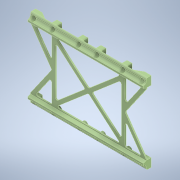
# Autodesk Inventor part: BodyStructure Centre
Saved by Autodesk Inventor 2022.2 (Build 262287030, 287C)
## iProperties
Created: 2019-11-07
Part Number: BodyStructure Centre
Material: solidworks materials|ABS
Document SubType Name: Modeling
Designer: Jochen
Density: 1.02 g/cm^3
Appearance: 151,157,178
Sending System: SolidWorks 2017
Last Author: Felix
Last Saved: 2021-02-23
Author: Jochen
Autodesk Inventor part; units mm, degrees
ref_plane "YZ Plane" through (0, 0, 0) normal (1, 0, 0) x (0, 1, 0)
ref_plane "XZ Plane" through (0, 0, 0) normal (0, 1, 0) x (-1, 0, 0)
ref_plane "Work Plane1" through (0, 0, 30) normal (0, 0, 1) x (1, 0, 0)
sketch "Sketch1" plane through (0, 0, 30) normal (0, 0, 1) x (1, 0, 0)
  line L0 (-80, -55) -> (80, -55)
  line L1 (80, 55) -> (-80, 55)
  line L2 (80, 42) -> (80, 42)
  line L3 (0, -77.5799) -> (0, 77.5799) construction
  line L4 (-112, 0) -> (112, 0) construction
  line L5 (-50.649, -42) -> (-50.649, -8.7287)
  line L6 (-45.649, 35.4185) -> (-45.649, -35.4185)
  line L7 (-50.649, -8.7287) -> (-73.9001, -42)
  line L8 (-80, -42) -> (-50.649, 0)
  line L9 (50.649, -8.7287) -> (73.9001, -42)
  line L10 (50.649, -42) -> (50.649, -8.7287)
  line L11 (45.649, 35.4185) -> (45.649, -35.4185)
  line L12 (80, -42) -> (50.649, 0)
  line L13 (50.649, 8.7287) -> (73.9001, 42)
  line L14 (80, 42) -> (50.649, 0)
  line L15 (50.649, 0) -> (50.649, 0)
  line L16 (50.649, 8.7287) -> (50.649, 42)
  line L17 (-50.649, 0) -> (-50.649, 0)
  line L18 (-80, 42) -> (-50.649, 0)
  line L19 (-50.649, 8.7287) -> (-73.9001, 42)
  line L20 (-80, 42) -> (-80, 42)
  line L21 (-50.649, 8.7287) -> (-50.649, 42)
  line L22 (73.9001, 42) -> (50.649, 42)
  line L23 (-73.9001, 42) -> (-50.649, 42)
  line L24 (-45.649, 42) -> (45.649, 42)
  line L25 (-80, -42) -> (-80, -42)
  line L26 (-50.649, -42) -> (-73.9001, -42)
  line L27 (45.649, -42) -> (-45.649, -42)
  line L28 (80, -42) -> (80, -42)
  line L29 (73.9001, -42) -> (50.649, -42)
  line L30 (80, -55) -> (80, -42)
  line L31 (80, 42) -> (80, 55)
  line L32 (-80, 55) -> (-80, 42)
  line L33 (-80, -42) -> (-80, -55)
  line L34 (-48.149, 55) -> (-48.149, -55) construction
  line L35 (-45.649, 42) -> (0, 2.9266)
  line L36 (0, 2.9266) -> (45.649, 42)
  line L37 (45.649, 35.4185) -> (4.2699, 0)
  line L38 (45.649, -35.4185) -> (4.2699, 0)
  line L39 (0, -2.9266) -> (45.649, -42)
  line L40 (-4.2699, 0) -> (-45.649, 35.4185)
  line L41 (-4.2699, 0) -> (-45.649, -35.4185)
  line L42 (0, -2.9266) -> (-45.649, -42)
  point P0 (0, 0)
  point P1 (-2.5, 42)
  point P2 (2.5, 42)
  point P3 (2.5, -42)
  point P4 (-2.5, -42)
  point P5 (50.649, 0)
  point P6 (-50.649, 0)
  dimension "d2" = 5
  dimension "d3" = 0
  dimension "d4" = 160
  dimension "d5" = 13
  dimension "d7" = 110
  dimension "d101" = 5
  dimension "d107" = 5
  constraints: 82 end point, 17 parallel, 15 collinear, 15 perpendicular, 11 point on line, 9 horizontal, 2 vertical, 19 other
  measures "d2" distance between parallel lines of L6 L5
  measures "d3" distance of L8.start L25.end
  measures "d4" distance of L0.start L0.end
  measures "d5" distance of L25.end L0.start
  measures "d7" distance between parallel lines of L1 L0
  measures "d101" distance between parallel lines of L8 L7
  measures "d107" distance between parallel lines of L42 L41
extrude "Extrusion1" add sketch "Sketch1" along normal blind 15.5
fillet "Fillet1" radius 2 22 edges at (-50.649, -42, 37.75) (-50.649, -8.7287, 37.75) (-73.9001, -42, 37.75) (-73.9001, 42, 37.75) (-50.649, 42, 37.75) (-50.649, 8.7287, 37.75) (50.649, -8.7287, 37.75) (50.649, -42, 37.75) (50.649, 42, 37.75) (50.649, 8.7287, 37.75) (73.9001, 42, 37.75) (73.9001, -42, 37.75) (-45.649, 35.4185, 37.75) (0, -2.9266, 37.75) (4.2699, 0, 37.75) (0, 2.9266, 37.75) (-4.2699, 0, 37.75) (-45.649, -35.4185, 37.75) (45.649, -35.4185, 37.75) (45.649, 35.4185, 37.75) (50.649, 0, 37.75) (-50.649, 0, 37.75)
fillet "Fillet1" radius 2 4 edges at (-45.649, 42, 37.75) (-45.649, -42, 37.75) (45.649, -42, 37.75) (45.649, 42, 37.75)
sketch "Sketch3" plane through (0, 0, 0) normal (1, 0, 0) x (0, 1, 0)
  line L0 (0, -10.1) -> (0, 60.6) construction
  line L1 (-77.5799, 0) -> (77.5799, 0) construction
  line L2 (-42, 45.5) -> (-55, 45.5) construction
  line L3 (-55, 45.5) -> (-42, 45.5) construction
  line L4 (-42, 45.5) -> (-1.1456, 45.5) construction
  line L5 (1.1456, 45.5) -> (42, 45.5) construction
  line L6 (42, 45.5) -> (55, 45.5) construction
  line L7 (55, 45.5) -> (42, 45.5) construction
  line L8 (42, 45.5) -> (1.1456, 45.5) construction
  line L9 (-1.1456, 45.5) -> (-42, 45.5) construction
  line L10 (13.9365, 45.5) -> (38.8544, 45.5) construction
  line L11 (42, 45.5) -> (38.8544, 45.5) construction
  line L12 (40, 45.5) -> (42, 45.5) construction
  line L13 (40, 45.5) -> (15.0821, 45.5) construction
  line L14 (13.9365, 45.5) -> (15.0821, 45.5) construction
  line L15 (15.0821, 45.5) -> (40, 45.5) construction
  line L16 (42, 45.5) -> (40, 45.5) construction
  line L17 (38.8544, 45.5) -> (42, 45.5) construction
  line L18 (38.8544, 45.5) -> (13.9365, 45.5) construction
  line L19 (15.0821, 45.5) -> (13.9365, 45.5) construction
  line L20 (-13.9365, 45.5) -> (-38.8544, 45.5) construction
  line L21 (-40, 45.5) -> (-42, 45.5) construction
  line L22 (-40, 45.5) -> (-15.0821, 45.5) construction
  line L23 (-13.9365, 45.5) -> (-15.0821, 45.5) construction
  line L24 (-38.8544, 45.5) -> (-42, 45.5) construction
  line L25 (-38.8544, 45.5) -> (-13.9365, 45.5) construction
  line L26 (-15.0821, 45.5) -> (-13.9365, 45.5) construction
  line L27 (-15.0821, 45.5) -> (-40, 45.5) construction
  line L28 (-42, 45.5) -> (-40, 45.5) construction
  line L29 (-42, 30) -> (-55, 30) construction
  line L30 (-1.1456, 30) -> (-42, 30) construction
  line L31 (42, 30) -> (1.1456, 30) construction
  line L32 (55, 30) -> (42, 30) construction
  line L33 (42, 30) -> (55, 30) construction
  line L34 (1.1456, 30) -> (42, 30) construction
  line L35 (-42, 30) -> (-1.1456, 30) construction
  line L36 (-55, 30) -> (-42, 30) construction
  line L37 (15.0821, 30) -> (13.9365, 30) construction
  line L38 (40, 30) -> (15.0821, 30) construction
  line L39 (42, 30) -> (40, 30) construction
  line L40 (38.8544, 30) -> (42, 30) construction
  line L41 (13.9365, 30) -> (38.8544, 30) construction
  line L42 (13.9365, 30) -> (15.0821, 30) construction
  line L43 (38.8544, 30) -> (13.9365, 30) construction
  line L44 (42, 30) -> (38.8544, 30) construction
  line L45 (40, 30) -> (42, 30) construction
  line L46 (15.0821, 30) -> (40, 30) construction
  line L47 (-15.0821, 30) -> (-13.9365, 30) construction
  line L48 (-40, 30) -> (-15.0821, 30) construction
  line L49 (-42, 30) -> (-40, 30) construction
  line L50 (-13.9365, 30) -> (-38.8544, 30) construction
  line L51 (-40, 30) -> (-42, 30) construction
  line L52 (-15.0821, 30) -> (-40, 30) construction
  line L53 (-13.9365, 30) -> (-15.0821, 30) construction
  line L54 (-38.8544, 30) -> (-13.9365, 30) construction
  line L55 (-42, 30) -> (-38.8544, 30) construction
  line L56 (55, 30) -> (55, 45.5) construction
  line L57 (55, 30) -> (55, 45.5) construction
  line L58 (-55, 30) -> (-55, 45.5) construction
  line L59 (-55, 30) -> (-55, 45.5) construction
  line L60 (-37, 30) -> (-37, 45.5) construction
  line L61 (-37, 30) -> (-37, 45.5) construction
  line L62 (-55, 30) -> (-55, 39.5)
  line L63 (-53, 41.5) -> (-48.9559, 41.5)
  line L64 (-48.9559, 41.5) -> (-47.5, 45.5)
  line L65 (-47.5, 45.5) -> (-45, 45.5)
  line L66 (-45, 45.5) -> (-43.5441, 41.5)
  line L67 (-43.5441, 41.5) -> (43.5441, 41.5)
  line L68 (43.5441, 41.5) -> (45, 45.5)
  line L69 (45, 45.5) -> (47.5, 45.5)
  line L70 (47.5, 45.5) -> (48.9559, 41.5)
  line L71 (55, 39.5) -> (55, 30)
  line L72 (55, 30) -> (-55, 30)
  line L73 (-46.25, 45.5) -> (-46.25, 30) construction
  line L74 (53, 41.5) -> (48.9559, 41.5)
  arc A0 (-53, 41.5) -> (-55, 39.5) centre (-53, 39.5) ccw
  arc A1 (55, 39.5) -> (53, 41.5) centre (53, 39.5) ccw
  line L75 (-38.8544, 30) -> (-42, 30) projected
  line L76 (-42, 45.5) -> (-38.8544, 45.5) projected
  line L77 (-47.5, 50.5) -> (-45, 50.5)
  line L78 (-45, 50.5) -> (-43.5441, 41.5)
  line L79 (-48.9559, 41.5) -> (-47.5, 50.5)
  line L80 (42, 45.5) -> (42, 30) projected
  line L81 (42, 30) -> (42, 45.5) projected
  line L82 (1.1456, 30) -> (-1.1456, 30) projected
  line L83 (-1.1456, 30) -> (1.1456, 30) projected
  line L84 (1.1456, 45.5) -> (-1.1456, 45.5) projected
  line L85 (-1.1456, 45.5) -> (1.1456, 45.5) projected
  point P0 (0, 0)
  point P1 (-55, 34.75)
  point P2 (50, 33)
  point P3 (48, 35)
  point P4 (-46.25, 50.5)
  dimension "d28" = 110
  dimension "d29" = 2.5
  dimension "d30" = 4
  dimension "d37" = 10
  dimension "d38" = 2
  dimension "d84" = 5
  constraints: 32 end point, 7 point on line, 4 parallel, 4 point on circle, 4 tangent, 3 collinear, 3 midpoint, 3 perpendicular, 2 centre point, 2 horizontal, 1 equal radius, 1 vertical, 5 other
  measures "d28" angle of L64 L65
  measures "d29" distance of L64.end L65.end
  measures "d30" distance between parallel lines of L63 L65
  measures "d37" distance from line of L58 L65.end
  measures "d38" radius of A0
  measures "d84" distance from line of point (-46.25, 50.5) L2
extrude "Extrusion3" cut sketch "Sketch3" along normal through all both and the other way through all contours L62 A0 L63 L64 L65 L66 L67 L80 L72 | L80 L67 L68 L69 L70 L74 A1 L71 L72 keep common part
sketch "Sketch12" plane through (80, -55, 30) normal (1, 0, 0) x (0, 0, -1)
  arc A0 (-11.5, 2) -> (-9.5, 0) centre (-9.5, 2) ccw projected
  line L0 (-11.5, 2) -> (-11.5, 6.0441) projected
  line L1 (-11.5, 6.0441) -> (-15.5, 7.5) projected
  line L2 (-15.5, 7.5) -> (-15.5, 10) projected
  line L3 (-15.5, 10) -> (-11.5, 11.4559) projected
  line L4 (-11.5, 11.4559) -> (-11.5, 13) projected
  line L5 (0, 13) -> (0, 0) projected
  line L6 (0, 0) -> (-9.5, 0) projected
  line L7 (-11.5, 97) -> (-11.5, 98.5441) projected
  line L8 (-11.5, 98.5441) -> (-15.5, 100) projected
  line L9 (-15.5, 100) -> (-15.5, 102.5) projected
  line L10 (-15.5, 102.5) -> (-11.5, 103.9559) projected
  line L11 (-11.5, 103.9559) -> (-11.5, 108) projected
  arc A1 (-9.5, 110) -> (-11.5, 108) centre (-9.5, 108) ccw projected
  line L12 (-9.5, 110) -> (0, 110) projected
  line L13 (0, 110) -> (0, 97) projected
  line L14 (-11.5, 6.0441) -> (-11.5, 2) projected
  line L15 (-11.5, 6.0441) -> (-11.5, 11.4559)
  line L16 (-11.5, 98.5441) -> (-11.5, 103.9559)
  line L17 (-11.5, 13) -> (0, 13) projected
  line L18 (0, 97) -> (-11.5, 97) projected
  point P0 (30, 55)
  constraints: 4 end point, 2 collinear
sketch "Sketch5" plane through (0, 0, 0) normal (0, 1, 0) x (-1, 0, 0)
  line L0 (114, 0) -> (-124, 0) construction
  line L1 (0, -9.1) -> (0, 54.6) construction
  line L2 (80, 41.5) -> (80, 45.5) construction
  line L3 (80, 45.5) -> (-90, 45.5) construction
  line L4 (-80, 30) -> (-80, 39.5) construction
  line L5 (-80, 30) -> (80, 30) construction
  line L6 (80, 30) -> (80, 39.5) construction
  line L7 (80, 39.5) -> (80, 41.5) construction
  line L8 (-80, 41.5) -> (-80, 39.5) construction
  line L9 (80, 39.5) -> (-80, 39.5) construction
  line L10 (-71, 34.5) -> (-61.4737, 40)
  line L11 (-61.4737, 40) -> (-52, 40)
  line L12 (-52, 40) -> (-52, 33)
  line L13 (-52, 33) -> (-45, 33)
  line L14 (-45, 33) -> (-45, 40)
  line L15 (-45, 40) -> (-16, 40)
  line L16 (-16, 40) -> (-16, 33)
  line L17 (-16, 33) -> (-9, 33)
  line L18 (-9, 33) -> (-9, 40)
  line L19 (-9, 40) -> (9, 40)
  line L20 (9, 40) -> (9, 33)
  line L21 (9, 33) -> (16, 33)
  line L22 (16, 33) -> (16, 40)
  line L23 (16, 40) -> (45, 40)
  line L24 (45, 40) -> (45, 33)
  line L25 (45, 33) -> (52, 33)
  line L26 (52, 33) -> (52, 40)
  line L27 (52, 40) -> (61.4737, 40)
  line L28 (61.4737, 40) -> (71, 34.5)
  line L29 (80, 34.5) -> (80, 45.5)
  line L30 (80, 30) -> (-80, 30) construction
  line L31 (80, 45.5) -> (-90, 45.5)
  line L32 (-90, 45.5) -> (-90, 34.5)
  line L33 (80, 41.5) -> (-80, 41.5) projected
  line L34 (80, 39.5) -> (-80, 39.5) projected
  line L35 (71, 34.5) -> (80, 34.5)
  line L36 (-90, 34.5) -> (-71, 34.5)
  line L37 (52, 40) -> (45, 40) construction
  line L38 (80, 39.5) -> (-80, 39.5) construction
  line L39 (-80, 45.5) -> (80, 45.5) construction
  point P0 (0, 0)
  point P1 (56.7369, 40)
  point P2 (48.5, 33)
  dimension "d44" = 30
  dimension "d47" = 7
  dimension "d48" = 9
  dimension "d49" = 5.5
  dimension "d51" = 11
  dimension "d52" = 9
  dimension "d96" = 7
  dimension "d102" = 48.5
  constraints: 54 end point, 15 point on line, 11 perpendicular, 4 collinear, 4 parallel, 2 midpoint, 1 vertical, 4 other
  measures "d44" angle of L5 L28
  measures "d47" distance between parallel lines of L26 L24
  measures "d48" distance between parallel lines of L1 L20
  measures "d49" distance from line of L3 point (56.737, 40)
  measures "d51" distance from line of L2.end L35
  measures "d52" distance of L28.end L29.start
  measures "d96" distance between parallel lines of L25 L37
  measures "d102" distance from line of L1 point (48.5, 33)
extrude "Extrusion5" cut sketch "Sketch5" along normal through all both and the other way through all contours L36 L32 L31 L29 L34 L28 L27 L26 L24 L23 L22 L20 L19 L18 L16 L15 L14 L12 L11 L10 | L34 L14 L13 L12 | L34 L18 L17 L16 | L29 L35 L28 L34 | L34 L22 L21 L20 | L26 L25 L24 L34 keep common part
sketch "Sketch6" plane through (0, 0, 0) normal (1, 0, 0) x (0, 1, 0)
  line L0 (0, -9.1) -> (0, 54.6) construction
  line L1 (-77.5799, 0) -> (77.5799, 0) construction
  line L2 (-38.535, 41.5) -> (-36.9915, 41.5) construction
  line L3 (-46.25, 40) -> (-46.25, 25)
  line L4 (-46.25, 25) -> (46.25, 25)
  line L5 (46.25, 25) -> (46.25, 40)
  line L6 (-46.25, 40) -> (46.25, 40)
  line L7 (-54.9365, 40) -> (54.9365, 40) projected
  line L8 (-45, 45.5) -> (-47.5, 45.5) construction
  line L9 (46.25, 25) -> (53.5, 25)
  line L10 (53.5, 25) -> (53.5, 40)
  line L11 (46.25, 40) -> (53.5, 40)
  line L12 (-46.25, 40) -> (-53.5, 40)
  line L13 (-53.5, 40) -> (-53.5, 25)
  line L14 (-53.5, 25) -> (-46.25, 25)
  line L15 (55, 33) -> (55, 39.5) projected
  line L16 (55, 33) -> (55, 25)
  line L17 (55, 25) -> (53.5, 25)
  line L18 (55, 33) -> (55, 40)
  line L19 (55, 40) -> (53.5, 40)
  line L20 (-53.5, 25) -> (-55, 25)
  line L21 (-55, 25) -> (-55, 40)
  line L22 (-55, 40) -> (-53.5, 40)
  point P0 (0, 0)
  point P1 (-46.25, 32.5)
  point P2 (42, 40)
  point P3 (-46.25, 45.5)
  point P4 (-55, 33)
  dimension "d75" = 1.5
  dimension "d104" = 15
  dimension "d106" = 7.25
  constraints: 36 end point, 7 point on line, 6 perpendicular, 4 collinear, 2 horizontal, 2 midpoint, 2 vertical, 1 parallel, 1 other
  measures "d75" distance between parallel lines of L6 L2
  measures "d104" distance from line of L6 L3.end
  measures "d106" distance between parallel lines of L5 L10
extrude "Extrusion6" cut sketch "Sketch6" along normal mid plane 140 contours L6 L5 L4 L3
sketch "Sketch9" plane through (45, -54.9365, 40) normal (0, 0, -1) x (-1, 0, 0)
  line L0 (-25, 91.3557) -> (-9.2884, 68.873) projected
  arc A0 (-9.2884, 68.873) -> (-5.649, 70.0186) centre (-7.649, 70.0186) ccw projected
  arc A1 (-5.649, 94.9365) -> (-7.649, 96.9365) centre (-7.649, 94.9365) ccw projected
  line L1 (-7.649, 96.9365) -> (-25, 96.9365) projected
  line L2 (-6.4496, 56.0821) -> (-25, 82.6269) projected
  line L3 (-35, 96.9365) -> (-35, 109.873) projected
  line L4 (-25, 82.6269) -> (-35, 96.9365) projected
  line L5 (-25, 27.2461) -> (-6.4496, 53.7909) projected
  line L6 (-35, 0) -> (-35, 12.9365) projected
  line L7 (-35, 12.9365) -> (-25, 27.2461) projected
  line L8 (125, 96.9365) -> (115, 82.6269) projected
  line L9 (125, 109.873) -> (125, 96.9365) projected
  line L10 (115, 27.2461) -> (125, 12.9365) projected
  line L11 (125, 12.9365) -> (125, 0) projected
  arc A2 (-5.649, 39.8543) -> (-9.2884, 41) centre (-7.649, 39.8543) ccw projected
  line L12 (-9.2884, 41) -> (-25, 18.5173) projected
  line L13 (-25, 12.9365) -> (-7.649, 12.9365) projected
  arc A3 (-7.649, 12.9365) -> (-5.649, 14.9365) centre (-7.649, 14.9365) ccw projected
  circle A4 centre (-30, 104.9365) radius 1.5
  circle A5 centre (32.5, 104.9365) radius 1.5
  circle A6 centre (-3.5, 104.9365) radius 1.5
  circle A7 centre (57.5, 104.9365) radius 1.5
  circle A8 centre (93.5, 104.9365) radius 1.5
  circle A9 centre (120, 104.9365) radius 1.5
  circle A10 centre (120, 4.9365) radius 1.5
  circle A11 centre (93.5, 4.9365) radius 1.5
  circle A12 centre (57.5, 4.9365) radius 1.5
  circle A13 centre (-3.5, 4.9365) radius 1.5
  circle A14 centre (32.5, 4.9365) radius 1.5
  circle A15 centre (-30, 4.9365) radius 1.5
  line L14 (-30, 104.9365) -> (120, 104.9365) construction
  line L15 (120, 104.9365) -> (120, 4.9365) construction
  line L16 (120, 4.9365) -> (-30, 4.9365) construction
  line L17 (-30, 4.9365) -> (-30, 104.9365) construction
  line L18 (157, 54.9365) -> (-67, 54.9365) construction
  line L19 (45, -22.6434) -> (45, 132.5164) construction
  line L20 (32.5, 104.9365) -> (32.5, 4.9365) construction
  line L21 (-3.5, 4.9365) -> (-3.5, 104.9365) construction
  line L22 (93.5, 104.9365) -> (93.5, 4.9365) construction
  line L23 (57.5, 104.9365) -> (57.5, 4.9365) construction
  circle A16 centre (-30, 4.9365) radius 2.9
  circle A17 centre (-3.5, 4.9365) radius 2.9
  circle A18 centre (32.5, 4.9365) radius 2.9
  circle A19 centre (57.5, 4.9365) radius 2.9
  circle A20 centre (93.5, 4.9365) radius 2.9
  circle A21 centre (120, 4.9365) radius 2.9
  circle A22 centre (120, 104.9365) radius 2.9
  circle A23 centre (93.5, 104.9365) radius 2.9
  circle A24 centre (57.5, 104.9365) radius 2.9
  circle A25 centre (32.5, 104.9365) radius 2.9
  circle A26 centre (-3.5, 104.9365) radius 2.9
  circle A27 centre (-30, 104.9365) radius 2.9
  line L24 (125, 0) -> (106.4737, 0) projected
  line L25 (-35, 109.873) -> (-16.4737, 109.873) projected
  line L26 (106.4737, 109.873) -> (125, 109.873) projected
  line L27 (-16.4737, 0) -> (-35, 0) projected
  line L28 (116.7018, 16.0821) -> (115, 18.5173) projected
  line L29 (115, 91.3557) -> (116.7018, 93.7909) projected
  line L30 (-26.7018, 93.7909) -> (-25, 91.3557) projected
  line L31 (-25, 18.5173) -> (-26.7018, 16.0821) projected
  line L32 (-5.649, 14.9365) -> (-5.649, 39.8543) projected
  line L33 (61, 8.6865) -> (61, 0) projected
  line L34 (106.4737, 0) -> (106.4737, 8.6865) projected
  line L35 (115, 18.5173) -> (115, 27.2461) projected
  line L36 (-16.4737, 109.873) -> (-16.4737, 101.1865) projected
  line L37 (95.649, 39.8543) -> (95.649, 14.9365) projected
  line L38 (97, 109.873) -> (97, 101.1865) projected
  line L39 (90, 101.1865) -> (90, 109.873) projected
  line L40 (54, 101.1865) -> (54, 109.873) projected
  line L41 (36, 109.873) -> (36, 101.1865) projected
  line L42 (29, 101.1865) -> (29, 109.873) projected
  line L43 (0, 109.873) -> (0, 101.1865) projected
  line L44 (-7, 101.1865) -> (-7, 109.873) projected
  line L45 (96.4496, 53.7909) -> (115, 27.2461) projected
  line L46 (115, 82.6269) -> (96.4496, 56.0821) projected
  line L47 (99.2884, 68.873) -> (115, 91.3557) projected
  line L48 (97.649, 12.9365) -> (115, 12.9365) projected
  line L49 (115, 18.5173) -> (99.2884, 41) projected
  line L50 (-25, 27.2461) -> (-25, 18.5173) projected
  line L51 (-25.0624, 12.9365) -> (-25, 12.9365) projected
  arc A28 (-26.7018, 16.0821) -> (-25.0624, 12.9365) centre (-25.0624, 14.9365) ccw projected
  line L52 (-25, 8.6865) -> (-16.4737, 8.6865) projected
  line L53 (-25, 12.9365) -> (-25, 8.6865) projected
  line L54 (-25, 91.3557) -> (-25, 82.6269) projected
  arc A29 (-25.0624, 96.9365) -> (-26.7018, 93.7909) centre (-25.0624, 94.9365) ccw projected
  line L55 (-25, 96.9365) -> (-25.0624, 96.9365) projected
  line L56 (-5.649, 70.0186) -> (-5.649, 94.9365) projected
  line L57 (-7, 8.6865) -> (0, 8.6865) projected
  line L58 (29, 8.6865) -> (36, 8.6865) projected
  line L59 (54, 8.6865) -> (61, 8.6865) projected
  line L60 (90, 8.6865) -> (97, 8.6865) projected
  line L61 (106.4737, 8.6865) -> (115, 8.6865) projected
  line L62 (115, 8.6865) -> (115, 12.9365) projected
  line L63 (115, 12.9365) -> (115.0624, 12.9365) projected
  arc A30 (115.0624, 12.9365) -> (116.7018, 16.0821) centre (115.0624, 14.9365) ccw projected
  line L64 (115, 82.6269) -> (115, 91.3557) projected
  arc A31 (116.7018, 93.7909) -> (115.0624, 96.9365) centre (115.0624, 94.9365) ccw projected
  line L65 (115.0624, 96.9365) -> (115, 96.9365) projected
  line L66 (115, 96.9365) -> (97.649, 96.9365) projected
  arc A32 (97.649, 96.9365) -> (95.649, 94.9365) centre (97.649, 94.9365) ccw projected
  line L67 (95.649, 94.9365) -> (95.649, 70.0186) projected
  arc A33 (95.649, 70.0186) -> (99.2884, 68.873) centre (97.649, 70.0186) ccw projected
  line L68 (-16.4737, 101.1865) -> (-25, 101.1865) projected
  line L69 (-25, 101.1865) -> (-25, 96.9365) projected
  arc A34 (99.2884, 41) -> (95.649, 39.8543) centre (97.649, 39.8543) ccw projected
  line L70 (115, 96.9365) -> (115, 101.1865) projected
  line L71 (115, 101.1865) -> (106.4737, 101.1865) projected
  line L72 (97, 101.1865) -> (90, 101.1865) projected
  line L73 (61, 101.1865) -> (54, 101.1865) projected
  line L74 (36, 101.1865) -> (29, 101.1865) projected
  line L75 (0, 101.1865) -> (-7, 101.1865) projected
  line L76 (-16.4737, 8.6865) -> (-16.4737, 0) projected
  line L77 (-7, 0) -> (-16.4737, 0) projected
  line L78 (-7, 0) -> (-7, 8.6865) projected
  line L79 (0, 8.6865) -> (0, 0) projected
  line L80 (29, 0) -> (0, 0) projected
  line L81 (29, 0) -> (29, 8.6865) projected
  line L82 (36, 8.6865) -> (36, 0) projected
  line L83 (54, 0) -> (36, 0) projected
  line L84 (54, 0) -> (54, 8.6865) projected
  line L85 (90, 0) -> (61, 0) projected
  line L86 (90, 0) -> (90, 8.6865) projected
  line L87 (97, 8.6865) -> (97, 0) projected
  line L88 (106.4737, 0) -> (97, 0) projected
  line L89 (0, 0) -> (-7, 0) projected
  line L90 (36, 0) -> (29, 0) projected
  line L91 (61, 0) -> (54, 0) projected
  line L92 (97, 0) -> (90, 0) projected
  line L93 (97, 109.873) -> (106.4737, 109.873) projected
  line L94 (90, 109.873) -> (97, 109.873) projected
  line L95 (61, 109.873) -> (90, 109.873) projected
  line L96 (54, 109.873) -> (61, 109.873) projected
  line L97 (36, 109.873) -> (54, 109.873) projected
  line L98 (29, 109.873) -> (36, 109.873) projected
  line L99 (0, 109.873) -> (29, 109.873) projected
  line L100 (-7, 109.873) -> (0, 109.873) projected
  line L101 (-16.4737, 109.873) -> (-7, 109.873) projected
  line L102 (106.4737, 101.1865) -> (106.4737, 109.873) projected
  line L103 (61, 109.873) -> (61, 101.1865) projected
  arc A35 (95.649, 14.9365) -> (97.649, 12.9365) centre (97.649, 14.9365) ccw projected
  line L104 (86.5373, 16.4559) -> (46.3005, 50.8966) projected
  line L105 (43.6995, 50.8966) -> (3.4627, 16.4559) projected
  arc A36 (3.4627, 16.4559) -> (4.7632, 12.9365) centre (4.7632, 14.9365) ccw projected
  line L106 (4.7632, 12.9365) -> (85.2368, 12.9365) projected
  arc A37 (85.2368, 12.9365) -> (86.5373, 16.4559) centre (85.2368, 14.9365) ccw projected
  line L107 (85.2368, 96.9365) -> (4.7632, 96.9365) projected
  arc A38 (4.7632, 96.9365) -> (3.4627, 93.4171) centre (4.7632, 94.9365) ccw projected
  line L108 (3.4627, 93.4171) -> (43.6995, 58.9763) projected
  line L109 (46.3005, 58.9763) -> (86.5373, 93.4171) projected
  arc A39 (86.5373, 93.4171) -> (85.2368, 96.9365) centre (85.2368, 94.9365) ccw projected
  line L110 (51.0451, 53.4171) -> (87.3485, 22.3431) projected
  arc A40 (87.3485, 22.3431) -> (90.649, 23.8625) centre (88.649, 23.8625) ccw projected
  line L111 (90.649, 23.8625) -> (90.649, 86.0105) projected
  arc A41 (90.649, 86.0105) -> (87.3485, 87.5299) centre (88.649, 86.0105) ccw projected
  line L112 (87.3485, 87.5299) -> (51.0451, 56.4559) projected
  arc A42 (51.0451, 56.4559) -> (51.0451, 53.4171) centre (52.3456, 54.9365) ccw projected
  line L113 (38.9549, 56.4559) -> (2.6515, 87.5299) projected
  arc A43 (2.6515, 87.5299) -> (-0.649, 86.0105) centre (1.351, 86.0105) ccw projected
  line L114 (-0.649, 86.0105) -> (-0.649, 23.8625) projected
  arc A44 (-0.649, 23.8625) -> (2.6515, 22.3431) centre (1.351, 23.8625) ccw projected
  line L115 (2.6515, 22.3431) -> (38.9549, 53.4171) projected
  arc A45 (38.9549, 53.4171) -> (38.9549, 56.4559) centre (37.6544, 54.9365) ccw projected
  arc A46 (43.6995, 58.9763) -> (46.3005, 58.9763) centre (45, 60.4957) ccw projected
  arc A47 (46.3005, 50.8966) -> (43.6995, 50.8966) centre (45, 49.3772) ccw projected
  arc A48 (-6.4496, 53.7909) -> (-6.4496, 56.0821) centre (-8.089, 54.9365) ccw projected
  arc A49 (96.4496, 56.0821) -> (96.4496, 53.7909) centre (98.089, 54.9365) ccw projected
  point P0 (45, 54.9365)
  point P1 (42.5, 12.9365)
  point P2 (-6, 80.6486)
  point P3 (-6, 19.2244)
  point P4 (-6, 14.9365)
  point P5 (47.5, 86.9365)
  point P6 (42.5, 76.9365)
  point P7 (42.5, 22.9365)
  point P8 (47.5, 76.9365)
  point P9 (47.5, 22.9365)
  point P10 (-6, 36.0374)
  point P11 (98.4175, 46.8521)
  point P12 (45, 52.0098)
  point P13 (45, 57.8631)
  point P14 (-5.649, 54.9365)
  point P15 (95.649, 54.9365)
  dimension "d61" = 3
  dimension "d63" = 100
  dimension "d64" = 75
  dimension "d65" = 48.5
  dimension "d66" = 12.5
  dimension "d69" = 5.8
  constraints: 24 centre point, 22 equal radius, 16 end point, 15 coincident, 8 point on line, 3 perpendicular, 2 parallel, 1 horizontal, 1 vertical, 7 other
  measures "d61" diameter of A4
  measures "d63" distance of L16.end L14.start
  measures "d64" distance from line of A15.centre L19
  measures "d65" distance from line of L21.start L19
  measures "d66" distance from line of L20.end L19
  measures "d69" diameter of A16
fillet "Fillet5" radius 3.5 18 edges at (-52, -46.25, 36.5) (-45, -46.25, 36.5) (-16, -46.25, 36.5) (-9, -46.25, 36.5) (0, -48.9559, 41.5) (9, -46.25, 36.5) (16, -46.25, 36.5) (45, -46.25, 36.5) (52, -46.25, 36.5) (52, 46.25, 36.5) (45, 46.25, 36.5) (16, 46.25, 36.5) (9, 46.25, 36.5) (-9, 46.25, 36.5) (-16, 46.25, 36.5) (-45, 46.25, 36.5) (-52, 46.25, 36.5) (0, 48.9559, 41.5)
fillet "Fillet4" radius 1 40 edges at (10.0251, 47.2751, 40) (12.5, 46.25, 40) (14.9749, 47.2751, 40) (9, 52.3432, 40) (9, -52.3432, 40) (16, 52.3432, 40) (16, -52.3432, 40) (46.0251, 47.2751, 40) (48.5, 46.25, 40) (50.9749, 47.2751, 40) (45, 52.3432, 40) (45, -52.3432, 40) (52, 52.3432, 40) (52, -52.3432, 40) (-48.5, 46.25, 40) (-46.0251, 47.2751, 40) (-50.9749, 47.2751, 40) (-52, 52.3432, 40) (-52, -52.3432, 40) (-45, 52.3432, 40) (-45, -52.3432, 40) (-16, 52.3432, 40) (-16, -52.3432, 40) (-9, 52.3432, 40) (-9, -52.3432, 40) (-14.9749, 47.2751, 40) (-12.5, 46.25, 40) (-10.0251, 47.2751, 40) (50.9749, -47.2751, 40) (46.0251, -47.2751, 40) (48.5, -46.25, 40) (10.0251, -47.2751, 40) (12.5, -46.25, 40) (14.9749, -47.2751, 40) (-14.9749, -47.2751, 40) (-12.5, -46.25, 40) (-10.0251, -47.2751, 40) (-50.9749, -47.2751, 40) (-48.5, -46.25, 40) (-46.0251, -47.2751, 40)
extrude "Extrusion8" cut sketch "Sketch9" along normal through all both and the other way through all contours A4 | A5 | A6 | A7 | A8 | A9 | A10 | A11 | A12 | A13 | A14 | A15
extrude "Extrusion9" cut sketch "Sketch9" along normal blind 1 and the other way blind 30 contours A4 | A5 | A6 | A7 | A8 | A9 | A10 | A11 | A12 | A13 | A14 | A15 | A16 | A17 | A18 | A19 | A20 | A21 | A22 | A23 | A24 | A25 | A26 | A27
sketch "Sketch10" plane through (0, 0, 0) normal (1, 0, 0) x (0, 1, 0)
  line L0 (-77.5799, 0) -> (77.5799, 0) construction
  line L1 (0, -9.1) -> (0, 54.6) construction
  line L2 (-43.5, 40) -> (43.5, 40)
  line L3 (43.5, 40) -> (43.5, 34.5)
  line L4 (43.5, 34.5) -> (-43.5, 34.5)
  line L5 (-43.5, 34.5) -> (-43.5, 40)
  line L6 (29.1214, 34.5) -> (55, 34.5) construction
  line L7 (-49.75, 40) -> (-54.9365, 40) construction
  point P0 (0, 0)
  dimension "d105" = 87
  constraints: 8 end point, 2 parallel, 1 collinear, 1 horizontal, 1 perpendicular, 1 point on line, 1 other
  measures "d105" distance of L3.end L4.end
extrude "Extrusion10" cut sketch "Sketch10" along normal through all both and the other way through all
equation "\"d2\" = d1"
equation "\"d1\" = 5"
body "Solid1"
body "Solid2"
